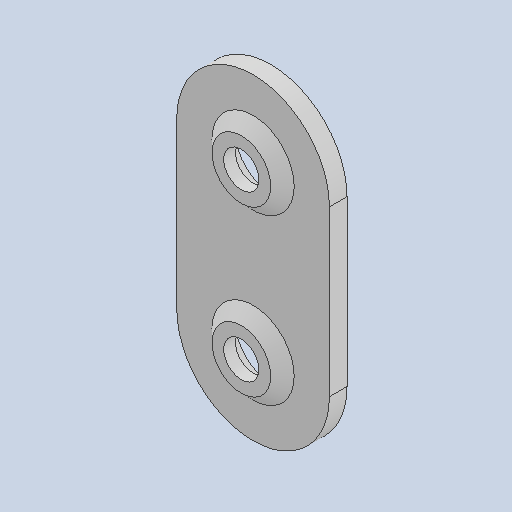
# Autodesk Inventor part: Belt Retainer
Saved by Autodesk Inventor 2022 (Build 260153000, 153)
## iProperties
Created: 2022-04-23
Part Number: Belt Retainer
Material: Generic
Document SubType Name: Modeling
Designer: Administrator
Density: 1 g/cm^3
Appearance: Default
Mass: 0.476025 g
Surface Area: 7.82991 cm^2
Volume: 0.476025 cm^3
Title: Component15
Author: Administrator
Autodesk Inventor part; units mm, degrees
ref_plane "YZ Plane" through (0, 0, 0) normal (1, 0, 0) x (0, 1, 0)
ref_plane "XZ Plane" through (0, 0, 0) normal (0, 1, 0) x (-1, 0, 0)
ref_plane "Work Plane1" through (0, 0, -15.5) normal (0, 0, 1) x (1, 0, 0)
sketch "Sketch1" plane through (0, 0, -15.5) normal (0, 0, 1) x (1, 0, 0)
  arc A0 (3.2082, 10) -> (16.2082, 10) centre (9.7082, 10) ccw
  line L0 (16.2082, 24) -> (16.2082, 10)
  line L1 (3.2082, 10) -> (3.2082, 24)
  arc A1 (16.2082, 24) -> (3.2082, 24) centre (9.7082, 24) ccw
  constraints: 4 end point, 4 point on circle, 2 centre point, 2 vertical, 1 equal radius, 1 parallel
extrude "Extrusion3" add sketch "Sketch1" along normal blind 1.5
sketch "Sketch2" plane through (0, 0, -14) normal (0, 0, 1) x (1, 0, 0)
  circle A0 centre (9.7082, 10) radius 2.5
  constraints: 1 centre point
extrude "Extrusion2" add sketch "Sketch2" along normal blind 1
sketch "Sketch3" plane through (0, 0, -14) normal (0, 0, 1) x (1, 0, 0)
  circle A0 centre (9.7082, 24) radius 2.5
  constraints: 1 centre point
extrude "Extrusion1" add sketch "Sketch3" along normal blind 1
hole "Hole2" at (9.7082, 10, -15.5) direction (0, 0, 1) diameter 3 depth 2.5
sketch "Sketch4" plane through (0, 0, -15.5) normal (0, 0, 1) x (1, 0, 0)
  point P0 (9.7082, 10)
hole "Hole1" at (9.7082, 24, -15.5) direction (0, 0, 1) diameter 3 depth 2.5
chamfer "Chamfer1" distance 1.5 angle 45 2 edges at (9.7082, 22.5, -15.5) (9.7082, 8.5, -15.5)
chamfer "Chamfer2" distance 1 angle 45 2 edges at (7.2082, 24, -14) (7.2082, 10, -14)
sketch "Sketch5" plane through (0, 0, -15.5) normal (0, 0, 1) x (1, 0, 0)
  point P0 (9.7082, 24)
body "Solid3"
